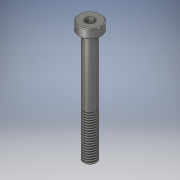
# Autodesk Inventor part: Bolt_M4x0.7_35mm_LSH
Saved by Autodesk Inventor 2018 (Build 220112000, 112)
## iProperties
Manager: Bradley
Created: 2016-07-03
Part Number: Bolt_M4x0.7_35mm_LSH
Material: Stainless Steel
Document SubType Name: Modeling
Designer: Bradley
Density: 8 g/cm^3
Appearance: Semi-Polished
Author: Bradley
Autodesk Inventor part; units mm, degrees
ref_plane "YZ Plane" through (0, 0, 0) normal (1, 0, 0) x (0, 1, 0)
ref_plane "XZ Plane" through (0, 0, 0) normal (0, 1, 0) x (-1, 0, 0)
ref_plane "XY Plane" through (0, 0, 0) normal (0, 0, 1) x (1, 0, 0)
sketch "Sketch1" plane through (0, 0, 0) normal (0, 0, 1) x (1, 0, 0)
  line L0 (0, 18.9) -> (0, -18.9)
  line L1 (0, -18.9) -> (1.75, -18.9)
  line L2 (1.75, -18.9) -> (2, -18.65)
  line L3 (2, -18.65) -> (2, 16)
  line L4 (2.1, 16.1) -> (3.25, 16.1)
  line L5 (3.5, 16.35) -> (3.5, 18.65)
  line L6 (3.25, 18.9) -> (0, 18.9)
  arc A0 (2.1, 16.1) -> (2, 16) centre (2.1, 16) ccw
  line L7 (3.25, 18.9) -> (3.5, 18.65)
  line L8 (3.25, 16.1) -> (3.5, 16.35)
  point P0 (0, 0)
  point P1 (3.5, 16.1)
  point P2 (3.5, 18.9)
  point P3 (0, 0)
  dimension "d0" = 7
  dimension "d1" = 2.8
  dimension "d3" = 4
  dimension "d4" = 4.2
  dimension "d5" = 135
  dimension "d6" = 0.25
  dimension "d7" = 35
  dimension "d9" = 0.25
  constraints: 18 end point, 6 perpendicular, 4 point on line, 2 point on circle, 2 tangent, 1 centre point, 1 coincident, 1 midpoint, 1 parallel, 1 vertical, 1 vertical alignment
  measures "d0" diameter of L5 L0
  measures "d1" distance of point (3.5, 16.1) point (3.5, 18.9)
  measures "d3" diameter of L3 L0
  measures "d4" diameter of L4.start L0
  measures "d5" angle of L3 L2
  measures "d6" horizontal distance of L1.end L2.end
  measures "d7" distance between parallel lines of L1 L4
  measures "d9" distance of L6.start point (3.5, 18.9)
revolve "Revolution1" add sketch "Sketch1" angle 360 about axis through (0, 18.9, 0) along (0, -1, 0)
sketch "Sketch2" plane through (0, 18.9, 0) normal (0, 1, 0) x (1, 0, 0)
  line L0 (0, -1.4434) -> (-1.25, -0.7217)
  line L1 (-1.25, -0.7217) -> (-1.25, 0.7217)
  line L2 (-1.25, 0.7217) -> (0, 1.4434)
  line L3 (0, 1.4434) -> (1.25, 0.7217)
  line L4 (1.25, 0.7217) -> (1.25, -0.7217)
  line L5 (1.25, -0.7217) -> (0, -1.4434)
  point P0 (0, 0)
  point P1 (0, 0)
  dimension "d11" = 2.5
  constraints: 12 end point, 1 coincident, 1 vertical, 13 other
  measures "d11" distance between parallel lines of L4 L1
extrude "Extrusion1" cut sketch "Sketch2" against normal blind 1.5
thread "Thread1" size "M4x0.7" class "6g" standard "ANSI Metric M Profile" length 14
sketch "Sketch3" plane through (0, 0, 0) normal (1, 0, 0) x (0, 1, 0)
  line L0 (18.9, 1.4434) -> (17.9, 0.4434)
  line L1 (17.9, 0.4434) -> (18.9, 0.4434)
  line L2 (18.9, 0.4434) -> (18.9, 1.4434)
  line L3 (-1.4, 0) -> (8.4, 0) projected
  point P0 (0, 0)
  dimension "d18" = 1
  constraints: 6 end point, 2 perpendicular, 1 vertical
  measures "d18" distance of L1.end L0.start
revolve "Revolution2" cut sketch "Sketch3" angle 360 about axis through (0, -10, 0) along (0, 1, 0)
body "Solid1"
